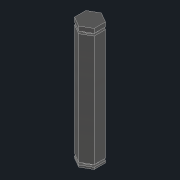
# Autodesk Inventor part: Wasp Omni Wheel Axle
Saved by Autodesk Inventor 2022 (Build 260153000, 153)
## iProperties
Created: 2022-09-18
Part Number: Wasp Omni Wheel Axle
Material: Generic
Document SubType Name: Modeling
Designer: robpl
Density: 1 g/cm^3
Appearance: Dark Gray
Author: robpl
Autodesk Inventor part; units mm, degrees
ref_plane "YZ Plane" through (0, 0, 0) normal (1, 0, 0) x (0, 1, 0)
ref_plane "XZ Plane" through (0, 0, 0) normal (0, 1, 0) x (-1, 0, 0)
ref_plane "XY Plane" through (0, 0, 0) normal (0, 0, 1) x (1, 0, 0)
sketch "Sketch1" plane through (0, 0, 0) normal (0, 1, 0) x (-1, 0, 0)
  line L0 (-6.35, 3.6662) -> (0, 7.3323)
  line L1 (0, 7.3323) -> (6.35, 3.6662)
  line L2 (6.35, 3.6662) -> (6.35, -3.6662)
  line L3 (6.35, -3.6662) -> (0, -7.3323)
  line L4 (0, -7.3323) -> (-6.35, -3.6662)
  line L5 (-6.35, -3.6662) -> (-6.35, 3.6662)
  point P0 (0, 0)
  point P1 (0, 0)
  dimension "d0" = 12.7
  constraints: 12 end point, 1 coincident, 1 vertical, 13 other
  measures "d0" distance between parallel lines of L2 L5
extrude "Extrusion1" add sketch "Sketch1" along normal blind 77
sketch "Sketch2" plane through (0, 0, 0) normal (1, 0, 0) x (0, 1, 0)
  line L0 (2.5, 15) -> (1, 15)
  line L1 (1, 15) -> (1, 5)
  line L2 (1, 5) -> (2.5, 5)
  line L3 (2.5, 5) -> (2.5, 15)
  line L4 (0, -3.6662) -> (0, 3.6662) projected
  line L5 (-15.24, 0) -> (91.44, 0) projected
  line L6 (74.5, 15) -> (76, 15)
  line L7 (76, 15) -> (76, 5)
  line L8 (76, 5) -> (74.5, 5)
  line L9 (74.5, 5) -> (74.5, 15)
  point P0 (0, 0)
  point P1 (0, 0)
  dimension "d3" = 1.5
  dimension "d4" = 10
  dimension "d5" = 5
  dimension "d6" = 1
  dimension "d15" = 72
  constraints: 16 end point, 4 parallel, 2 equal length, 2 horizontal, 2 perpendicular, 1 coincident, 1 horizontal alignment
  measures "d3" distance of L0.start L0.end
  measures "d4" distance of L0.end L1.end
  measures "d5" distance from line of L2 point (0, 0)
  measures "d6" distance between parallel lines of L4 L1
  measures "d15" distance between parallel lines of L3 L9
revolve "Revolution1" cut sketch "Sketch2" angle 360 about axis through (0, -10, 0) along (0, 1, 0)
body "Solid1"
